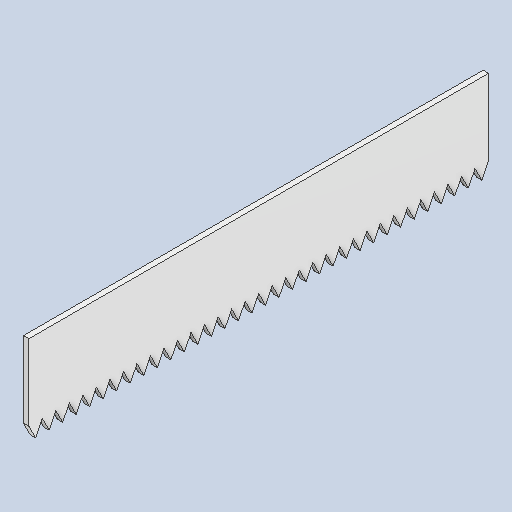
# Autodesk Inventor part: Blade
Saved by Autodesk Inventor 2022 (Build 260153000, 153)
## iProperties
Created: 2022-03-31
Part Number: Blade
Material: UHMW, White
Document SubType Name: Modeling
Designer: mpate
Density: 0.94 g/cm^3
Appearance: Smooth - White
Author: mpate
Autodesk Inventor part; units mm, degrees
ref_plane "YZ Plane" through (0, 0, 0) normal (1, 0, 0) x (0, 1, 0)
ref_plane "XZ Plane" through (0, 0, 0) normal (0, 1, 0) x (-1, 0, 0)
sketch "Sketch1" plane through (0, 0, 0) normal (0, 1, 0) x (-1, 0, 0)
  line L0 (0, 0) -> (2, 0)
  line L1 (2, 0) -> (2, -170)
  line L2 (2, -170) -> (0, -170)
  line L3 (0, -170) -> (0, 0)
  dimension "d0" = 2
  dimension "d1" = 170
  constraints: 8 end point, 2 parallel, 1 horizontal, 1 perpendicular
  measures "d0" distance between parallel lines of L1 L3
  measures "d1" distance between parallel lines of L0 L2
extrude "Extrusion1" add sketch "Sketch1" along normal blind 28
ref_plane "Work Plane1" through (0, -5, 0) normal (0, -1, 0) x (1, 0, 0)
sketch "Sketch6" plane through (0, 0, 0) normal (1, 0, 0) x (0, 0, -1)
  line L0 (170, 0) -> (0, 0) projected
  line L1 (0, 0) -> (2.5, -5)
  line L2 (2.5, -5) -> (5, 0)
  line L3 (204, -5) -> (-34, -5) projected
  dimension "d5" = 2.5
  dimension "d6" = 2.5
  dimension "d7" = 0
  constraints: 4 end point, 1 point on line
  measures "d5" horizontal distance of L0.end L1.end
  measures "d6" horizontal distance of L1.end L2.end
  measures "d7" distance from line of L3 L1.end
extrude "Extrusion2" add sketch "Sketch6" against normal blind 2
pattern_linear "Rectangular Pattern1" count 34 spacing 5 along (0, 0, -1) of "Extrusion2"
body "Solid1"
